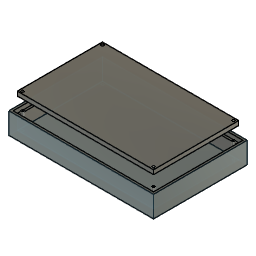
Modelo 3d da case (Autodesk Fusion 360 design; units mm, degrees)
Autodesk Fusion 360 part; units mm, degrees
note: some values were not read from the file. Chosen so that the rebuilt part matches the saved one: which bodies a step acts on.
sketch "Esboço1" plane through (0, 0, 0) normal (0, 0, 1) x (1, 0, 0)
  line L0 (0, 0) -> (170, 0)
  line L1 (170, 0) -> (170, 110)
  line L2 (170, 110) -> (0, 110)
  line L3 (0, 110) -> (0, 0)
  dimension "d1" = 170
  dimension "d2" = 110
  dimension "d3" = 170
  dimension "d4" = 110
  constraint coincident L0.start L3.end
  constraint horizontal L0
  constraint perpendicular L0 L1
  constraint perpendicular L1 L2
  constraint perpendicular L2 L3
  measures "d1" distance of L0.start L0.end
  measures "d2" distance of L0.end L1.end
  measures "d3" distance of L1.end L2.end
  measures "d4" distance of L2.end L0.start
extrude "Extrusão1" add sketch "Esboço1" along normal blind 5 makes body 1
sketch "Esboço2" plane through (0, 0, 5) normal (0, 0, 1) x (-1, 0, 0)
  line L0 (0, -110) -> (0, 0)
  line L1 (0, 0) -> (-170, 0)
  line L2 (-170, 0) -> (-170, -110)
  line L3 (-170, -110) -> (0, -110)
  line L4 (-85, -105) -> (-170, -105)
  line L5 (-85, -105) -> (0, -105)
  line L6 (0, -105) -> (0, -110)
  line L7 (0, -110) -> (-170, -110)
  line L8 (-170, -110) -> (-170, -105)
  constraint coincident L2 L4.end
  constraint perpendicular L2 L4
  constraint coincident L0 L5.end
  constraint perpendicular L0 L5
  constraint coincident L0.start L3.end
  constraint coincident L2.end L3.start
extrude "Extrusão2" add sketch "Esboço2" along normal blind 20 contours L0 L2 L3 L4 L5 L6 L7 L8 bodies 1
sketch "Esboço3" plane through (0, 0, 0) normal (0, 1, 0) x (1, 0, 0)
sketch "Esboço4" plane through (0, 0, 5) normal (0, 0, 1) x (-1, 0, 0)
  line L0 (-170, -105) -> (0, -105)
  line L1 (0, -105) -> (0, 0)
  line L2 (0, 0) -> (-170, 0)
  line L3 (-170, 0) -> (-170, -105)
  line L4 (-90, -5) -> (-85, -5)
  line L5 (-85, -5) -> (0, -5)
  line L6 (-90, -5) -> (-170, -5)
  line L7 (-170, -5) -> (-170, 0)
  line L8 (-170, 0) -> (0, 0)
  line L9 (0, 0) -> (0, -5)
  constraint coincident L1 L5.end
  constraint perpendicular L1 L5
  constraint coincident L3 L6.end
  constraint perpendicular L3 L6
  constraint coincident L2.end L3.start
  constraint coincident L1.end L2.start
extrude "Extrusão3" add sketch "Esboço4" along normal blind 20 contours L1 L2 L3 L4 L5 L6 L7 L8 L9 bodies 1
sketch "Esboço5" plane through (0, 0, 5) normal (0, 0, 1) x (-1, 0, 0)
  line L0 (0, -5) -> (-170, -5)
  line L1 (-170, -5) -> (-170, -105)
  line L2 (-170, -105) -> (0, -105)
  line L3 (0, -105) -> (0, -5)
  line L4 (-165, -55) -> (-165, -5)
  line L5 (-165, -5) -> (-170, -5)
  line L6 (-170, -5) -> (-170, -105)
  line L7 (-170, -105) -> (-165, -105)
  line L8 (-165, -55) -> (-165, -105)
  dimension "d14" = 5
  constraint coincident L0 L4.end
  constraint perpendicular L0 L4
  constraint coincident L0.end L1.start
  constraint coincident L1.end L2.start
  constraint perpendicular L6 L7
  measures "d14" distance of L1.end L7.end
extrude "Extrusão4" add sketch "Esboço5" along normal blind 20 contours L0 L1 L2 L4 L5 L6 L7 L8 bodies 1
sketch "Esboço6" plane through (0, 0, 0) normal (1, 0, 0) x (0, 1, 0)
sketch "Esboço7" plane through (0, 0, 5) normal (0, 0, 1) x (-1, 0, 0)
  line L0 (-165, -5) -> (-165, -105)
  line L1 (-165, -105) -> (0, -105)
  line L2 (0, -105) -> (0, -5)
  line L3 (0, -5) -> (-165, -5)
  line L4 (-5, -55) -> (-5, -105)
  line L5 (-5, -55) -> (-5, -5)
  line L6 (-5, -5) -> (0, -5)
  line L7 (0, -5) -> (0, -105)
  line L8 (0, -105) -> (-5, -105)
  constraint coincident L1 L4.end
  constraint perpendicular L1 L4
  constraint coincident L3 L5.end
  constraint perpendicular L3 L5
  constraint coincident L2.end L3.start
  constraint coincident L1.end L2.start
extrude "Extrusão5" add sketch "Esboço7" along normal blind 20 contours L1 L2 L3 L4 L5 L6 L7 L8 bodies 1
sketch "Esboço8" plane through (0, 0, 5) normal (0, 0, 1) x (-1, 0, 0)
  line L0 (-5, -105) -> (-5, -5)
  line L1 (-5, -5) -> (-165, -5)
  line L2 (-165, -5) -> (-165, -105)
  line L3 (-165, -105) -> (-5, -105)
  line L4 (-5.5, -2.5) -> (-85, -2.5)
  line L5 (-2.5, -4) -> (-2.5, -2.5)
  line L6 (-5.5, -2.5) -> (-2.5, -2.5)
  line L7 (-2.5, -4) -> (-2.5, -65)
  line L8 (-2.5, -105) -> (-2.5, -82)
  line L9 (-2.5, -81.75) -> (-2.5, -82)
  line L10 (-2.5, -65) -> (-2.5, -81.75)
  line L11 (-6, -107.5) -> (-2.5, -107.5)
  line L12 (-2.5, -105) -> (-2.5, -107.5)
  line L13 (-167.5, -104) -> (-167.5, -107.5)
  line L14 (-166, -107.5) -> (-167.5, -107.5)
  line L15 (-167.5, -7) -> (-167.5, -2.5)
  line L16 (-164, -2.5) -> (-167.5, -2.5)
  line L17 (-164, -2.5) -> (-85, -2.5)
  line L18 (-167.5, -7) -> (-167.5, -104)
  line L19 (-166, -107.5) -> (-6, -107.5)
  constraint perpendicular L5 L6
  constraint perpendicular L11 L12
  constraint perpendicular L13 L14
  constraint perpendicular L15 L16
  constraint parallel L4 L17
  constraint perpendicular L17 L18
  constraint perpendicular L8 L19
sketch "Esboço9" plane through (0, 0, 0) normal (0, 1, 0) x (1, 0, 0)
sketch "Esboço10" plane through (0, 0, 5) normal (0, 0, 1) x (-1, 0, 0)
extrude "Extrusão6" add sketch "Esboço8" along normal blind 20 contours L0 L1 L2 L3 bodies 1
sketch "Esboço11" plane through (0, 0, 25) normal (0, 0, 1) x (-1, 0, 0)
  line L0 (0, -110) -> (0, 0)
  line L1 (0, 0) -> (-170, 0)
  line L2 (-170, 0) -> (-170, -110)
  line L3 (-170, -110) -> (0, -110)
  line L4 (-167.3, -2.5) -> (-167.5, -2.5)
  line L5 (-167.5, -3.0755) -> (-167.5, -2.5)
  line L6 (-167.5, -105.7811) -> (-167.5, -107.5)
  line L7 (-165.3442, -107.5) -> (-167.5, -107.5)
  line L8 (-167.5, -105.7811) -> (-167.5, -3.0755)
  line L9 (-2.5, -2.7808) -> (-2.5, -2.5)
  line L10 (-5, -2.5) -> (-2.5, -2.5)
  line L11 (-2.5, -2.7808) -> (-2.5, -6.5)
  line L12 (-5, -2.5) -> (-167.3, -2.5)
  line L13 (-5.0233, -107.5) -> (-2.5, -107.5)
  line L14 (-2.5, -101) -> (-2.5, -107.5)
  line L15 (-2.5, -101) -> (-2.5, -6.5)
  line L16 (-5.0233, -107.5) -> (-165.3442, -107.5)
  constraint horizontal L4
  constraint perpendicular L1 L8
  constraint perpendicular L9 L10
  constraint parallel L9 L11
  constraint perpendicular L13 L14
  constraint perpendicular L1 L15
  constraint perpendicular L6 L16
extrude "Extrusão7" cut sketch "Esboço11" against normal blind 5 contours L4 L5 L6 L7 L8 L9 L10 L11 L12 L13 L14 L15 L16 bodies 1
sketch "Esboço12" plane through (0, 0, 20) normal (0, 0, 1) x (-1, 0, 0)
  line L0 (-2.5, -107.5) -> (-2.5, -2.5)
  line L1 (-2.5, -2.5) -> (-5, -2.5)
  line L2 (-5, -2.5) -> (-167.3, -2.5)
  line L3 (-167.3, -2.5) -> (-167.5, -2.5)
  line L4 (-167.5, -2.5) -> (-167.5, -107.5)
  line L5 (-167.5, -107.5) -> (-2.5, -107.5)
  line L6 (-6.3584, -105) -> (-5, -105)
  line L7 (-5, -101.6689) -> (-5, -105)
  line L8 (-9.7477, -5) -> (-9.1031, -5)
  line L9 (-9.1031, -5) -> (-5, -5)
  line L10 (-5, -8.9989) -> (-5, -5)
  line L11 (-162.7335, -5) -> (-165, -5)
  line L12 (-165, -9.6115) -> (-165, -5)
  line L13 (-165, -101.8786) -> (-165, -105)
  line L14 (-161.9219, -105) -> (-165, -105)
  line L15 (-161.9219, -105) -> (-6.3584, -105)
  line L16 (-5, -101.6689) -> (-5, -8.9989)
  line L17 (-9.7477, -5) -> (-162.7335, -5)
  line L18 (-165, -9.6115) -> (-165, -101.8786)
  constraint perpendicular L6 L7
  constraint perpendicular L9 L10
  constraint perpendicular L13 L14
  constraint parallel L6 L15
  constraint perpendicular L1 L16
  constraint parallel L2 L17
  constraint perpendicular L14 L18
extrude "Extrusão8" cut sketch "Esboço12" against normal blind 15 contours L6 L7 L8 L9 L10 L11 L12 L13 L14 L15 L16 L17 L18 bodies 1
sketch "Esboço13" plane through (0, 0, 5) normal (0, 0, 1) x (-1, 0, 0)
  line L0 (-5, -5) -> (-165, -5)
  line L1 (-165, -5) -> (-165, -105)
  line L2 (-165, -105) -> (-5, -105)
  line L3 (-5, -105) -> (-5, -8.9989)
  line L4 (-5, -8.9989) -> (-5, -5)
  circle A0 centre (-162, -8) radius 1.45
  circle A1 centre (-8, -8) radius 1.45
  circle A2 centre (-8, -102) radius 1.45
  circle A3 centre (-162, -102) radius 1.45
  dimension "d60" = 2.9
  dimension "d63" = 2.9
  dimension "d66" = 2.9
  dimension "d69" = 2.9
  measures "d60" diameter of A0
  measures "d63" diameter of A1
  measures "d66" diameter of A2
  measures "d69" diameter of A3
extrude "Extrusão9" add sketch "Esboço13" along normal blind 15 contours A0 | A1 | A2 | A3 bodies 1
extrude "Extrusão10" add 1 faces at (160.9354, 101.8575, 20) along direction (0, 0, 1) blind 5 on bodies 1 bodies 1
extrude "Extrusão11" add 1 faces at (162.4544, 7.5494, 20) along direction (0, 0, 1) blind 5 on bodies 1 bodies 1
extrude "Extrusão12" add 1 faces at (8.3704, 8.5433, 20) along direction (0, 0, 1) blind 5 on bodies 1 bodies 1
extrude "Extrusão13" add 1 faces at (8.1076, 101.5288, 20) along direction (0, 0, 1) blind 5 on bodies 1 bodies 1
sketch "Esboço14" plane through (0, 0, 5) normal (0, 0, 1) x (-1, 0, 0)
  circle A0 centre (-8, -102) radius 1.45
  circle A1 centre (-8, -8) radius 1.45
  circle A2 centre (-162, -102) radius 1.45
  circle A3 centre (-162, -8) radius 1.45
  line L0 (-5, -5) -> (-165, -5)
  line L1 (-165, -105) -> (-5, -105)
  line L2 (-5, -105) -> (-5, -8.9989)
  line L3 (-5, -8.9989) -> (-5, -5)
  circle A4 centre (-85, -55) radius 20
  dimension "d84" = 40
  measures "d84" diameter of A4
extrude "Extrusão14" add sketch "Esboço14" along normal blind 40 contours A4 bodies 1
sketch "Esboço15" plane through (0, 0, 5) normal (0, 0, 1) x (-1, 0, 0)
  circle A0 centre (-8, -102) radius 1.45
  circle A1 centre (-8, -8) radius 1.45
  circle A2 centre (-162, -102) radius 1.45
  circle A3 centre (-162, -8) radius 1.45
  line L0 (-5, -5) -> (-165, -5)
  line L1 (-165, -5) -> (-165, -105)
  line L2 (-165, -105) -> (-5, -105)
  line L3 (-5, -105) -> (-5, -8.9989)
  line L4 (-5, -8.9989) -> (-5, -5)
sketch "Esboço16" plane through (0, 5, 0) normal (0, 1, 0) x (-1, 0, 0)
  line L0 (-5, 20) -> (-165, 20)
  line L1 (-165, 20) -> (-165, 5)
  line L2 (-165, 5) -> (-5, 5)
  line L3 (-5, 5) -> (-5, 20)
extrude "Extrusão15" cut 1 faces at (85.3995, 61.2157, 45) along direction (0, 0, -1) blind 40 on bodies 1 bodies 1
sketch "Esboço17" plane through (0, 0, 25) normal (0, 0, 1) x (-1, 0, 0)
  line L0 (-5, -2.5) -> (-2.5, -2.5)
  line L1 (-2.5, -2.5) -> (-2.5, -107.5)
  line L2 (-2.5, -107.5) -> (-167.5, -107.5)
  line L3 (-167.5, -107.5) -> (-167.5, -2.5)
  line L4 (-167.5, -2.5) -> (-167.3, -2.5)
  line L5 (-167.3, -2.5) -> (-5, -2.5)
  line L6 (0, -110) -> (0, 0)
  line L7 (0, 0) -> (-170, 0)
  line L8 (-170, 0) -> (-170, -110)
  line L9 (-170, -110) -> (0, -110)
sketch "Esboço18" plane through (170, 0, 0) normal (1, 0, 0) x (0, 1, 0)
  line L0 (0, 0) -> (110, 0)
  line L1 (110, 0) -> (110, 25)
  line L2 (110, 25) -> (0, 25)
  line L3 (0, 25) -> (0, 0)
sketch "Esboço19" plane through (0, 0, 0) normal (0, -1, 0) x (1, 0, 0)
  line L0 (0, 0) -> (170, 0)
  line L1 (170, 0) -> (170, 25)
  line L2 (170, 25) -> (0, 25)
  line L3 (0, 25) -> (0, 0)
sketch "Esboço20" plane through (0, 0, 0) normal (0, -1, 0) x (1, 0, 0)
sketch "Esboço21" plane through (170, 0, 0) normal (1, 0, 0) x (0, 1, 0)
sketch "Esboço22" plane through (0, 110, 0) normal (0, 1, 0) x (-1, 0, 0)
  line L0 (-170, 0) -> (0, 0)
  line L1 (0, 0) -> (0, 25)
  line L2 (0, 25) -> (-170, 25)
  line L3 (-170, 25) -> (-170, 0)
sketch "Esboço23" plane through (0, 0, 0) normal (-1, 0, 0) x (0, -1, 0)
  line L0 (-110, 0) -> (0, 0)
  line L1 (0, 0) -> (0, 25)
  line L2 (0, 25) -> (-110, 25)
  line L3 (-110, 25) -> (-110, 0)
extrude "Extrusão16" add sketch "Esboço17" along normal blind 20 bodies 1
sketch "Esboço24" plane through (0, 110, 0) normal (0, 1, 0) x (-1, 0, 0)
  line L0 (-170, 0) -> (0, 0)
  line L1 (0, 0) -> (0, 45)
  line L2 (0, 45) -> (-170, 45)
  line L3 (-170, 45) -> (-170, 0)
  line L4 (-170, 40) -> (0, 40)
  line L5 (0, 40) -> (0, 25)
  line L6 (0, 25) -> (-170, 25)
  line L7 (-170, 40) -> (-170, 25)
  dimension "d98" = 5
  dimension "d99" = 170
  dimension "d100" = 15
  dimension "d101" = 170
  constraint perpendicular L3 L4
  constraint perpendicular L4 L5
  constraint perpendicular L1 L6
  measures "d98" distance of L2.end L4.start
  measures "d99" distance of L4.start L4.end
  measures "d100" distance of L4.end L5.end
  measures "d101" distance of L5.end L6.end
extrude "Extrusão17" cut sketch "Esboço24" against normal blind 110 contours L1 L3 L4 L5 L6 L7 bodies 1 makes body 2 at (58.3333, 0.8333, 40)
extrude "Extrusão18" add 1 faces at (113.3333, 110, 41.6667) along direction (0, -1, 0) blind 110 on bodies 2 bodies 2
extrude "Extrusão19" cut 1 faces at (170, 36.6667, 41.6667) along direction (-1, 0, 0) blind 5 on bodies 2 bodies 2
extrude "Extrusão20" cut 1 faces at (55, 0, 41.6667) along direction (0, 1, 0) blind 5 on bodies 2 bodies 2
extrude "Extrusão21" cut 1 faces at (0, 75, 43.3333) along direction (1, 0, 0) blind 5 on bodies 2 bodies 2
extrude "Extrusão22" cut 1 faces at (111.6667, 110, 41.6667) along direction (0, -1, 0) blind 5 on bodies 2 bodies 2
sketch "Esboço25" plane through (0, 0, 45) normal (0, 0, 1) x (-1, 0, 0)
  line L0 (-165, -105) -> (-5, -105)
  line L1 (-5, -105) -> (-5, -5)
  line L2 (-5, -5) -> (-165, -5)
  line L3 (-165, -5) -> (-165, -105)
  circle A0 centre (-8, -102) radius 1.5
  circle A1 centre (-8, -8) radius 1.5
  circle A2 centre (-162, -8) radius 1.5
  circle A3 centre (-162, -102) radius 1.5
  dimension "d116" = 3
  dimension "d119" = 3
  dimension "d122" = 3
  dimension "d125" = 3
  measures "d116" diameter of A0
  measures "d119" diameter of A1
  measures "d122" diameter of A2
  measures "d125" diameter of A3
extrude "Extrusão23" cut sketch "Esboço25" against normal blind 10 contours A0 | A1 | A2 | A3 bodies 2
sketch "Esboço26" plane through (0, 0, 25) normal (0, 0, 1) x (-1, 0, 0)
  circle A0 centre (-8, -102) radius 1.45
  circle A1 centre (-8, -8) radius 0.5
  circle A2 centre (-162, -8) radius 0.5
  circle A3 centre (-162, -102) radius 0.5
  circle A4 centre (-8, -102) radius 0.5
  dimension "d128" = 1
  dimension "d129" = 1
  dimension "d130" = 1
  dimension "d131" = 1
  constraint concentric A0 A4
  measures "d128" diameter of A1
  measures "d129" diameter of A2
  measures "d130" diameter of A3
  measures "d131" diameter of A4
extrude "Extrusão24" cut sketch "Esboço26" against normal blind 10 contours A1 | A2 | A3 | A4 bodies 1
